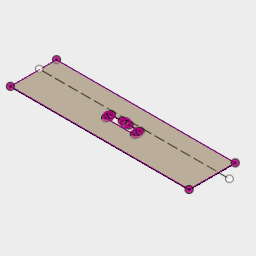
euroloch v3 (Autodesk Fusion 360 design; units mm, degrees)
Autodesk Fusion 360 part; units mm, degrees
sketch "Sketch1" plane through (0, 0, 0) normal (0, 1, 0) x (1, 0, 0)
  line L0 (2.5, -2.5) -> (27.5, -2.5)
  arc A0 (27.5, -2.5) -> (27.5, 2.5) centre (27.5, 0) ccw
  arc A1 (2.5, 2.5) -> (2.5, -2.5) centre (2.5, 0) ccw
  line L1 (0, 0) -> (30, 0) construction
  line L2 (15, 2.5) -> (15, 10) construction
  line L3 (15, 2.5) -> (15, -7) construction
  arc A2 (18, 2.5) -> (12, 2.5) centre (15, 2.5) ccw
  line L4 (27.5, 2.5) -> (18, 2.5)
  line L5 (12, 2.5) -> (2.5, 2.5)
  point P0 (15, 0)
  dimension "d2" = 6
  dimension "d3" = 30
  dimension "d5" = 5
  measures "d2" diameter of A2
  measures "d3" distance of L1.start L1.end
  measures "d5" distance of L0 L4
sketch "Sketch2" plane through (0, 0, 0) normal (0, 1, 0) x (1, 0, 0)
  line L0 (30, 10) -> (30, -30)
  line L1 (92.5, 20) -> (-62.5, 20)
  line L2 (-62.5, 20) -> (-62.5, -20)
  line L3 (-62.5, -20) -> (92.5, -20)
  line L4 (92.5, -20) -> (92.5, 20)
  line L5 (92.5, 20) -> (-62.5, -20) construction
  line L6 (-62.5, 20) -> (92.5, -20) construction
  point P0 (15, 0)
  point P1 (15, 0)
  dimension "d7" = 40
  dimension "d10" = 40
  dimension "d11" = 155
  measures "d7" distance of L0.start L0.end
  measures "d10" distance of L1.end L2.end
  measures "d11" distance of L2.end L3.end
extrude "Extrude1" add sketch "Sketch2" sketch "Sketch1" along normal blind 0.6 of sketch 2
extrude "Extrude2" cut sketch "Sketch1" along normal up to surface (0.6 mm away)
sketch "Sketch3" plane through (0, 0.6, 0) normal (0, 1, 0) x (-1, 0, 0)
  line L0 (-27.5, 2.5) -> (-2.5, 2.5)
  arc A0 (-2.5, -2.5) -> (-2.5, 2.5) centre (-2.5, 0) ccw
  line L1 (-2.5, -2.5) -> (-12, -2.5)
  arc A1 (-18, -2.5) -> (-12, -2.5) centre (-15, -2.5) ccw
  line L2 (-18, -2.5) -> (-27.5, -2.5)
  arc A2 (-27.5, 2.5) -> (-27.5, -2.5) centre (-27.5, 0) ccw
  line L3 (-92.5, 20) -> (-92.5, -20)
  line L4 (-92.5, -20) -> (62.5, -20)
  line L5 (62.5, -20) -> (62.5, 20)
  line L6 (62.5, 20) -> (-92.5, 20)
  line L7 (-2.5, 2.5) -> (-27.5, 2.5)
  arc A3 (-27.5, 2.5) -> (-27.5, -2.5) centre (-27.5, 0) ccw
  line L8 (-27.5, -2.5) -> (-18, -2.5)
  arc A4 (-18, -2.5) -> (-12, -2.5) centre (-15, -2.5) ccw
  line L9 (-12, -2.5) -> (-2.5, -2.5)
  arc A5 (-2.5, -2.5) -> (-2.5, 2.5) centre (-2.5, 0) ccw
  line L10 (-92.5, -20) -> (-92.5, 20)
  line L11 (-92.5, 20) -> (62.5, 20)
  line L12 (62.5, 20) -> (62.5, -20)
  line L13 (62.5, -20) -> (-92.5, -20)
  line L14 (-15, -5.5) -> (-102, -5.5) construction
  line L15 (-15, -5.5) -> (63, -5.5) construction
  dimension "d17" = 8
  measures "d17" distance of L0 L15
equation "d7 = höhe"
equation "breite = 155 mm"
equation "höhe = 40 mm"
equation "d10 = höhe"
equation "d11 = breite"
equation "dicke = 0.6 mm"
equation "d13 = dicke"
